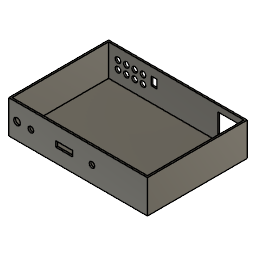
Amplifier Enclosure (Autodesk Fusion 360 design; units mm, degrees)
part number: 2026-03-23-19-31-45-976
Autodesk Fusion 360 part; units mm, degrees
sketch "Sketch1" plane through (0, 0, 0) normal (0, 0, 1) x (1, 0, 0)
  line L0 (-125, 90) -> (125, 90)
  line L1 (125, 90) -> (125, -90)
  line L2 (125, -90) -> (-125, -90)
  line L3 (-125, -90) -> (-125, 90)
  dimension "d1" = 250
  dimension "d2" = 180
  dimension "d3" = 90
  dimension "d4" = 125
  constraint horizontal L0
  constraint vertical L1
  constraint horizontal L2
  constraint vertical L3
  measures "d1" distance of L0.start L0.end
  measures "d2" distance of L0.start L2.end
  measures "d3" distance of origin L0
  measures "d4" distance of origin L3
extrude "Extrude1" add sketch "Sketch1" along normal blind 60
shell "Shell1" thickness 3 removed faces 1 at (-41.6667, 30, 60)
sketch "Sketch2" plane through (0, -90, 0) normal (0, -1, 0) x (1, 0, 0)
  line L0 (-125, 0) -> (125, 0)
  line L1 (125, 0) -> (125, 60)
  line L2 (125, 60) -> (-125, 60)
  line L3 (-125, 60) -> (-125, 0)
  circle A0 centre (-85, 30) radius 5
  circle A1 centre (25, 30) radius 5
  line L4 (-40, 35) -> (-10, 35)
  line L5 (-10, 35) -> (-10, 25)
  line L6 (-10, 25) -> (-40, 25)
  line L7 (-40, 25) -> (-40, 35)
  circle A2 centre (-110, 30) radius 6
  dimension "d8" = 10
  dimension "d9" = 10
  dimension "d10" = 12
  constraint horizontal L4
  constraint vertical L5
  constraint horizontal L6
  constraint vertical L7
  measures "d8" diameter of A0
  measures "d9" diameter of A1
  measures "d10" diameter of A2
extrude "Extrude2" cut sketch "Sketch2" against normal blind 10 contours A0 | A1 | L4 L5 L6 L7 | A2
sketch "Sketch3" plane through (0, 90, 0) normal (0, 1, 0) x (-1, 0, 0)
  line L0 (-125, 0) -> (125, 0)
  line L1 (125, 0) -> (125, 60)
  line L2 (125, 60) -> (-125, 60)
  line L3 (-125, 60) -> (-125, 0)
  circle A0 centre (105, 40) radius 5
  circle A1 centre (105, 25) radius 5
  circle A2 centre (90, 25) radius 5
  circle A3 centre (90, 40) radius 5
  circle A4 centre (105, 25) radius 5
  circle A5 centre (60, 25) radius 5
  circle A6 centre (75, 25) radius 5
  circle A7 centre (75, 25) radius 5
  circle A8 centre (75, 40) radius 5
  circle A9 centre (60, 40) radius 5
  line L4 (35, 45) -> (45, 45)
  line L5 (45, 45) -> (45, 30)
  line L6 (45, 30) -> (35, 30)
  line L7 (35, 30) -> (35, 45)
  line L8 (-110, 49) -> (-75, 49)
  line L9 (-75, 49) -> (-75, 14)
  line L10 (-75, 14) -> (-110, 14)
  line L11 (-110, 14) -> (-110, 49)
  dimension "d13" = 10
  dimension "d14" = 10
  dimension "d15" = 10
  dimension "d16" = 10
  dimension "d17" = 10
  dimension "d18" = 10
  dimension "d19" = 10
  dimension "d20" = 10
  dimension "d21" = 10
  dimension "d22" = 10
  constraint horizontal L4
  constraint vertical L5
  constraint horizontal L6
  constraint vertical L7
  constraint horizontal L8
  constraint vertical L9
  constraint horizontal L10
  constraint vertical L11
  measures "d13" diameter of A0
  measures "d14" diameter of A1
  measures "d15" diameter of A2
  measures "d16" diameter of A3
  measures "d17" diameter of A4
  measures "d18" diameter of A8
  measures "d19" diameter of A6
  measures "d20" diameter of A5
  measures "d21" diameter of A9
  measures "d22" diameter of A7
extrude "Extrude3" cut sketch "Sketch3" against normal blind 10 contours A0 | A1 A4 | A2 | A3 | A5 | A6 A7 | A8 | A9 | L4 L5 L6 L7 | L8 L9 L10 L11
